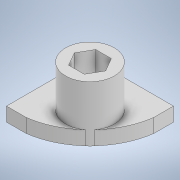
# Autodesk Inventor part: holder
Saved by Autodesk Inventor 2020 (Build 240168000, 168)
## iProperties
Created: 2022-08-25
Part Number: holder
Material: Типовые
Document SubType Name: Modeling
Designer: zigma
Density: 1 g/cm^3
Appearance: По умолчанию
Author: zigma
Autodesk Inventor part; units mm, degrees
ref_plane "YZ Plane" through (0, 0, 0) normal (1, 0, 0) x (0, 1, 0)
ref_plane "XZ Plane" through (0, 0, 0) normal (0, 1, 0) x (-1, 0, 0)
ref_plane "XY Plane" through (0, 0, 0) normal (0, 0, 1) x (1, 0, 0)
sketch "Эскиз1" plane through (0, 0, 0) normal (0, 1, 0) x (-1, 0, 0)
  line L0 (0, 0) -> (12, 0)
  line L1 (12, 0) -> (12, -12)
  line L2 (12, -12) -> (0, -12)
  line L3 (0, -12) -> (0, 0)
  dimension "d0" = 12
  dimension "d1" = 12
  constraints: 8 end point, 2 parallel, 1 horizontal, 1 perpendicular
  measures "d0" distance of L1.end L2.end
  measures "d1" distance of L0.end L1.end
extrude "Выдавливание1" add sketch "Эскиз1" along normal blind 2
sketch "Эскиз2" plane through (0, 2, 0) normal (0, 1, 0) x (1, 0, 0)
  line L0 (0, 12) -> (-12, 12) projected
  line L1 (0, 0) -> (0, 12) projected
  line L2 (-12, 12) -> (0, 12)
  line L3 (0, 12) -> (0, 0)
  line L4 (0, 0) -> (-12, 0)
  line L5 (-12, 0) -> (-12, 12)
  circle A0 centre (-5.5, 5.5) radius 5.5
  circle A1 centre (-5.5, 5.5) radius 3.5
  line L6 (-12, 12) -> (-12, 0) projected
  line L7 (-12, 11) -> (0, 11)
  line L8 (-11, 12) -> (-11, 0)
  line L9 (-12, 0) -> (0, 0) projected
  dimension "d5" = 7
  dimension "d19" = 1
  dimension "d20" = 1
  dimension "d21" = 11
  constraints: 12 end point, 4 point on line, 3 tangent, 2 centre point, 2 horizontal, 2 parallel, 1 coincident, 1 perpendicular, 1 vertical
  measures "d5" diameter of A1
  measures "d19" distance between parallel lines of L5 L8
  measures "d20" distance between parallel lines of L0 L7
  measures "d21" diameter of A0
extrude "Выдавливание2" add sketch "Эскиз2" along normal blind 6 contours A1
sketch "Эскиз3" plane through (-5.5, 8, -5.5) normal (0, 1, 0) x (1, 0, 0)
  circle A0 centre (0, 0) radius 3.5 projected
  circle A1 centre (0, 0) radius 1.5
  point P0 (5.5, -5.5)
  dimension "d8" = 3
  constraints: 1 centre point, 1 coincident
  measures "d8" diameter of A1
extrude "Выдавливание3" cut sketch "Эскиз3" against normal blind 8 contours A1
sketch "Эскиз5" plane through (-5.5, 8, -5.5) normal (0, 1, 0) x (1, 0, 0)
  circle A0 centre (0, 0) radius 1.5 projected
  circle A1 centre (0, 0) radius 2.25
  line L0 (2.25, 0) -> (1.125, -1.9486)
  line L1 (1.125, -1.9486) -> (-1.125, -1.9486)
  line L2 (-1.125, -1.9486) -> (-2.25, 0)
  line L3 (-2.25, 0) -> (-1.125, 1.9486)
  line L4 (-1.125, 1.9486) -> (1.125, 1.9486)
  line L5 (1.125, 1.9486) -> (2.25, 0)
  point P0 (5.5, -5.5)
  dimension "d14" = 4.5
  constraints: 12 end point, 2 coincident, 1 horizontal alignment, 15 other
extrude "Выдавливание5" cut sketch "Эскиз5" against normal blind 4 contours L0 L1 L2 L3 L4 L5
sketch "Эскиз6" plane through (0, 2, 0) normal (0, 1, 0) x (1, 0, 0)
  line L0 (-12, 0) -> (0, 0) projected
  line L1 (0, 0) -> (0, 12) projected
  line L2 (0, 12) -> (0, 0)
  line L3 (0, 0) -> (-12, 0)
  circle A0 centre (-5.5, 5.5) radius 3.5 projected
  arc A1 (-12, 0) -> (0, 12) centre (-10.599, 10.599) ccw
  point P0 (0, 9.1981)
  point P1 (-2.7251, 3.3669)
  point P2 (-3.3669, 2.7251)
  point P3 (-9.1981, 0)
  constraints: 4 end point, 2 perpendicular, 2 point on circle, 1 centre point
extrude "Выдавливание6" cut sketch "Эскиз6" against normal blind 4 contours A1 A0 L1 L0
